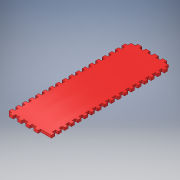
# Autodesk Inventor part: 000.204 - Боковая стенка управляющая
Saved by Autodesk Inventor 2019 (Build 230136000, 136)
## iProperties
Created: 2020-02-27
Part Number: 000.204 - Боковая стенка управляющая
Material: Типовые
Document SubType Name: Modeling
Designer: Петров Иван
Density: 1 g/cm^3
Appearance: Светло-красный
Author: Петров Иван
Autodesk Inventor part; units mm, degrees
ref_plane "YZ Plane" through (0, 0, 0) normal (1, 0, 0) x (0, 1, 0)
ref_plane "XZ Plane" through (0, 0, 0) normal (0, 1, 0) x (-1, 0, 0)
ref_plane "XY Plane" through (0, 0, 0) normal (0, 0, 1) x (1, 0, 0)
sketch "Эскиз1" plane through (0, 0, 0) normal (0, 1, 0) x (-1, 0, 0)
  line L0 (-22.5, 72) -> (22.5, 72)
  line L1 (22.5, 72) -> (22.5, -72)
  line L2 (22.5, -72) -> (-22.5, -72)
  line L3 (-22.5, -72) -> (-22.5, 72)
  line L4 (-22.5, 72) -> (22.5, -72) construction
  line L5 (22.5, 72) -> (-22.5, -72) construction
  point P0 (0, 0)
  point P1 (0, 0)
  dimension "d0" = 45
  dimension "d1" = 144
  constraints: 12 end point, 3 midpoint, 2 parallel, 1 horizontal, 1 perpendicular, 1 other
  measures "d0" distance of L1.end L2.end
  measures "d1" distance of L0.end L1.end
extrude "Выдавливание1" add sketch "Эскиз1" along normal blind 3
sketch "Эскиз2" plane through (0, 3, 0) normal (0, 1, 0) x (0, 0, -1)
  line L0 (-72, -22.5) -> (72, -22.5) projected
  line L1 (-72, -22.5) -> (-68, -22.5)
  line L2 (-68, -22.5) -> (-68, -25.5)
  line L3 (-68, -25.5) -> (-72, -25.5)
  line L4 (-72, -25.5) -> (-72, -22.5)
  point P0 (0, 0)
  dimension "d5" = 4
  dimension "d6" = 3
  constraints: 8 end point, 2 parallel, 1 horizontal, 1 perpendicular
  measures "d5" distance of L2.end L3.end
  measures "d6" distance of L1.end L2.end
extrude "Выдавливание2" add sketch "Эскиз2" against normal blind 3
pattern_linear "Прямоуг.массив1" count 18 spacing 8 along (0, 0, -1) of "Выдавливание2"
sketch "Эскиз3" plane through (0, 3, 0) normal (0, 1, 0) x (0, 0, -1)
  line L0 (72, 22.5) -> (-72, 22.5) projected
  line L1 (-72, 22.5) -> (-75, 22.5)
  line L2 (-75, 22.5) -> (-75, 17.5)
  line L3 (-75, 17.5) -> (-72, 17.5)
  line L4 (-72, 17.5) -> (-72, 22.5)
  line L5 (72, -22.5) -> (72, 22.5) projected
  line L6 (72, 17.5) -> (75, 17.5)
  line L7 (75, 17.5) -> (75, 12.5)
  line L8 (75, 12.5) -> (72, 12.5)
  line L9 (72, 12.5) -> (72, 17.5)
  point P0 (0, 0)
  dimension "d17" = 3
  dimension "d18" = 5
  dimension "d15" = 3
  dimension "d16" = 5
  dimension "d14" = 5
  constraints: 16 end point, 4 parallel, 2 horizontal, 2 perpendicular, 1 point on line
  measures "d17" distance of L3.end L2.end
  measures "d18" distance of L2.end L1.end
  measures "d15" distance of L7.end L8.end
  measures "d16" distance of L6.end L7.end
  measures "d14" distance between parallel lines of L0 L6
extrude "Выдавливание3" add sketch "Эскиз3" against normal blind 3
pattern_linear "Прямоуг.массив2" count 4 spacing 10 along (1, 0, 0) of "Выдавливание3"
mirror "Зеркальное отражение1" about plane through (0, 0, 0) normal (1, 0, 0) of "Выдавливание2", "Прямоуг.массив1"
